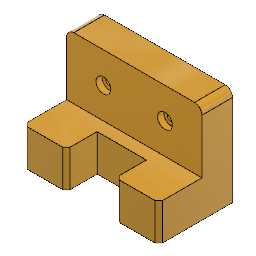
Task1a v0 (Autodesk Fusion 360 design; units mm, degrees)
Autodesk Fusion 360 part; units mm, degrees
sketch "Sketch1" plane through (0, 0, 0) normal (0, 1, 0) x (1, 0, 0)
sketch "Sketch2" plane through (0, 0, 0) normal (0, 1, 0) x (1, 0, 0)
  line L0 (0, 0) -> (35, 0)
  line L1 (35, 0) -> (35, 25)
  line L2 (35, 25) -> (75, 25)
  line L3 (75, 25) -> (75, 0)
  line L4 (75, 0) -> (110, 0)
  line L5 (110, 0) -> (110, 60)
  line L6 (110, 60) -> (0, 60)
  line L7 (0, 60) -> (0, 0)
  line L8 (-35, -3) -> (-35, -25)
  line L9 (-35, -3) -> (-35, -25)
  dimension "d1" = 35
  dimension "d2" = 25
  dimension "d3" = 40
  dimension "d4" = 25
  dimension "d5" = 35
  dimension "d7" = 60
  dimension "d8" = 110
  constraint coincident L0.start L7.end
  constraint horizontal L0
  constraint perpendicular L0 L1
  constraint perpendicular L1 L2
  constraint perpendicular L0 L3
  constraint perpendicular L3 L4
  constraint perpendicular L4 L5
  constraint perpendicular L5 L6
  measures "d1" distance of L0.start L0.end
  measures "d2" distance of L0.end L1.end
  measures "d3" distance of L1.end L2.end
  measures "d4" distance of L2.end L3.end
  measures "d5" distance of L3.end L4.end
  measures "d7" distance of L4.end L5.end
  measures "d8" distance of L5.end L6.end
extrude "Extrude1" add sketch "Sketch2" along normal blind 30
sketch "Sketch3" plane through (0, 30, 0) normal (0, 1, 0) x (-1, 0, 0)
  line L0 (0, -60) -> (0, 0)
  line L1 (0, 0) -> (-35, 0)
  line L2 (-35, 0) -> (-35, -25)
  line L3 (-35, -25) -> (-75, -25)
  line L4 (-75, -25) -> (-75, 0)
  line L5 (-75, 0) -> (-110, 0)
  line L6 (-110, 0) -> (-110, -60)
  line L7 (-110, -60) -> (0, -60)
  line L8 (0, -60) -> (-110, -60)
  line L9 (-110, -60) -> (-110, -35)
  line L10 (-110, -35) -> (0, -35)
  line L11 (0, -35) -> (0, -60)
  dimension "d11" = 25
  constraint horizontal L8
  constraint vertical L9
  constraint horizontal L10
  constraint vertical L11
  constraint coincident L0.start L7.end
  measures "d11" distance of L0.start L10.end
extrude "Extrude2" add sketch "Sketch3" along normal blind 50 contours L0 L6 L7 L8 L9 L10 L11
sketch "Sketch4" plane through (0, 0, -35) normal (0, 0, 1) x (1, 0, 0)
  line L0 (0, 30) -> (110, 30)
  line L1 (110, 30) -> (110, 80)
  line L2 (110, 80) -> (0, 80)
  line L3 (0, 80) -> (0, 30)
  circle A0 centre (30, 55) radius 6
  circle A1 centre (80, 55) radius 6
extrude "Extrude3" cut sketch "Sketch4" against normal blind 5 contours A0 | A1
sketch "Sketch5" plane through (0, 0, -40) normal (0, 0, 1) x (1, 0, 0)
  circle A0 centre (30, 55) radius 6
  circle A1 centre (30, 55) radius 3
  dimension "d21" = 6
  constraint concentric A0 A1
  measures "d21" diameter of A1
sketch "Sketch6" plane through (0, 0, -40) normal (0, 0, 1) x (1, 0, 0)
  circle A0 centre (80, 55) radius 6
  circle A1 centre (80, 55) radius 3
  dimension "d22" = 6
  constraint concentric A0 A1
  measures "d22" diameter of A1
extrude "Extrude4" cut sketch "Sketch5" sketch "Sketch6" against normal blind 50 contours A1 of sketch 2 contours A1
sketch "Sketch7" plane through (0, 0, -35) normal (0, 0, 1) x (1, 0, 0)
  circle A0 centre (80, 55) radius 6
  circle A1 centre (30, 55) radius 6
  line L0 (0, 30) -> (110, 30)
  line L1 (110, 30) -> (110, 80)
  line L2 (110, 80) -> (0, 80)
  line L3 (0, 80) -> (0, 30)
fillet "Fillet2" radius 6 1 edges at (110, 80, -47.5)
fillet "Fillet3" radius 6 1 edges at (0, 80, -47.5)
sketch "Sketch8" plane through (0, 30, 0) normal (0, 1, 0) x (-1, 0, 0)
  line L0 (-110, -35) -> (0, -35)
  line L1 (0, -35) -> (0, 0)
  line L2 (0, 0) -> (-35, 0)
  line L3 (-35, 0) -> (-35, -25)
  line L4 (-35, -25) -> (-75, -25)
  line L5 (-75, -25) -> (-75, 0)
  line L6 (-75, 0) -> (-110, 0)
  line L7 (-110, 0) -> (-110, -35)
  line L8 (0, 0) -> (0, -3) construction
  line L9 (0, -3) -> (-3, 0)
  line L10 (0, -3) -> (-4.2426, -3) construction
  line L11 (0, 0) -> (0, -3)
  line L12 (-17.5, 0) -> (-17.5, -4.7879) construction
  line L13 (-35, -3) -> (-32, 0)
  line L14 (-35, 0) -> (-35, -3)
  line L15 (-35, 0) -> (-35, -3) construction
  point P0 (-35, 0)
  point P1 (-35, 0)
  dimension "d28" = 3
  dimension "d29" = 45
  constraint coincident L1.end L2.start
  constraint perpendicular L2 L8
  constraint horizontal L10
  constraint coincident L2 L9.end
  constraint midpoint L2 L12.start
  constraint perpendicular L2 L12
  constraint symmetric L1.end L12 P1
  constraint symmetric L8.end L12 L13.start
  constraint symmetric L9.end L12 L13.end
  measures "d28" distance of L1.end L8.end
  measures "d29" angle of L9 L10
extrude "Extrude5" cut sketch "Sketch8" against normal blind 30 contours L1 L2 L9 L11 | L2 L3 L13 L14
sketch "Sketch10" plane through (0, 30, 0) normal (0, 1, 0) x (-1, 0, 0)
  line L0 (-32, 0) -> (-35, -3)
  line L1 (-35, -3) -> (-35, -25)
  line L2 (-35, -25) -> (-75, -25)
  line L3 (-75, -25) -> (-75, 0)
  line L4 (-75, 0) -> (-110, 0)
  line L5 (-110, 0) -> (-110, -35)
  line L6 (-110, -35) -> (0, -35)
  line L7 (0, -35) -> (0, -3)
  line L8 (0, -3) -> (-3, 0)
  line L9 (-3, 0) -> (-32, 0)
  line L10 (-110, 0) -> (-110, -3) construction
  line L11 (-110, -3) -> (-107, 0)
  line L12 (-110, -3) -> (-105.7574, -3) construction
  line L13 (-92.5, 0) -> (-92.5, -2.9277) construction
  line L14 (-75, -3) -> (-78, 0)
  line L15 (-75, 0) -> (-75, -3) construction
  line L16 (-75, -3) -> (-79.2426, -3) construction
  point P0 (-75, 0)
  dimension "d32" = 3
  dimension "d33" = 45
  constraint coincident L4.end L5.start
  constraint perpendicular L4 L10
  constraint horizontal L12
  constraint coincident L4 L11.end
  constraint midpoint L4 L13.start
  constraint perpendicular L4 L13
  constraint symmetric L4.end L13 P0
  constraint symmetric L10.end L13 L14.start
  constraint symmetric L11.end L13 L14.end
  constraint symmetric L12.end L13 L16.end
  measures "d32" distance of L4.end L10.end
  measures "d33" angle of L11 L12
extrude "Extrude6" cut sketch "Sketch10" against normal blind 30 contours L3 L4 L14 | L4 L5 L11
sketch "Sketch9" plane through (0, 30, 0) normal (0, 1, 0) x (-1, 0, 0)
  line L0 (-32, 0) -> (-35, -3)
  line L1 (-35, -3) -> (-35, -25)
  line L2 (-35, -25) -> (-75, -25)
  line L3 (-75, -25) -> (-75, 0)
  line L4 (-75, 0) -> (-110, 0)
  line L5 (-110, 0) -> (-110, -35)
  line L6 (-110, -35) -> (0, -35)
  line L7 (0, -35) -> (0, -3)
  line L8 (0, -3) -> (-3, 0)
  line L9 (-3, 0) -> (-32, 0)
  line L10 (-55, -25) -> (-55, -31.6762) construction
  constraint midpoint L2 L10.start
  constraint perpendicular L2 L10
fillet "Fillet1" [suppressed]
